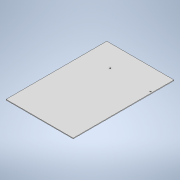
# Autodesk Inventor part: NewShooterBoard
Saved by Autodesk Inventor 2020 (Build 240168000, 168)
## iProperties
Created: 2021-04-22
Part Number: NewShooterBoard
Material: Generic
Document SubType Name: Modeling
Designer: tdmp4
Density: 1 g/cm^3
Appearance: Default
Author: tdmp4
Autodesk Inventor part; units mm, degrees
ref_plane "YZ Plane" through (0, 0, 0) normal (1, 0, 0) x (0, 1, 0)
ref_plane "XZ Plane" through (0, 0, 0) normal (0, 1, 0) x (-1, 0, 0)
ref_plane "XY Plane" through (0, 0, 0) normal (0, 0, 1) x (1, 0, 0)
sketch "Sketch1" plane through (0, 0, 0) normal (0, 1, 0) x (-1, 0, 0)
  line L0 (0, 0) -> (254, 0)
  line L1 (254, 0) -> (254, 381)
  line L2 (254, 381) -> (0, 381)
  line L3 (0, 381) -> (0, 0)
  dimension "d0" = 254
  dimension "d1" = 381
  constraints: 8 end point, 2 parallel, 1 horizontal, 1 perpendicular
  measures "d0" distance of L1.end L2.end
  measures "d1" distance of L2.end L0.start
extrude "Extrusion1" add sketch "Sketch1" along normal blind 2.54
sketch "Sketch2" plane through (0, 2.54, 0) normal (0, 1, 0) x (1, 0, 0)
  line L0 (0, -381) -> (0, 0) projected
  line L1 (0, 0) -> (0, -82.55)
  line L2 (0, -82.55) -> (-82.55, -82.55)
  circle A0 centre (-82.55, -82.55) radius 76.2
  circle A1 centre (-82.55, -82.55) radius 72.39
  circle A2 centre (-82.55, -82.55) radius 69.85
  circle A3 centre (-158.75, -82.55) radius 2.286
  circle A4 centre (-6.35, -82.55) radius 2.286
  dimension "d4" = 82.55
  dimension "d5" = 82.55
  dimension "d6" = 152.4
  dimension "d7" = 144.78
  dimension "d8" = 139.7
  dimension "d9" = 4.572
  dimension "d10" = 4.572
  constraints: 5 centre point, 4 end point, 3 coincident, 2 point on circle, 2 point on line, 1 perpendicular
  measures "d4" distance of L0.end L1.end
  measures "d5" distance of L1.end L2.end
  measures "d6" diameter of A0
  measures "d7" diameter of A1
  measures "d8" diameter of A2
  measures "d9" diameter of A3
  measures "d10" diameter of A4
extrude "Extrusion2" cut sketch "Sketch2" against normal blind 2.54 contours A4 A0 L2 | L2 A0 A4 | A0 A4 L2 | L2 A4 A0 | A3 A0 | A0 A3
body "Solid1"
